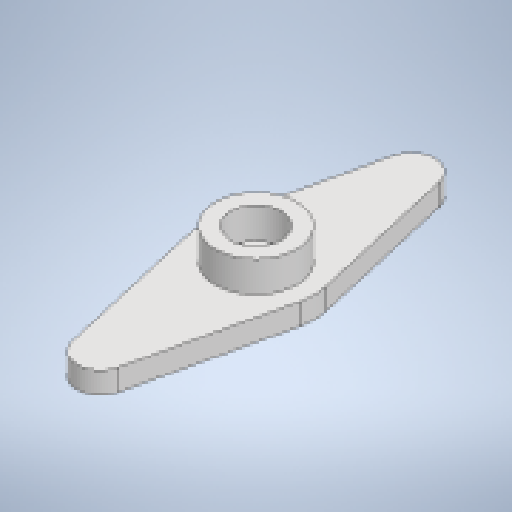
# Autodesk Inventor part: Brazo
Saved by Autodesk Inventor 2024 (Build 280153000, 153)
## iProperties
Created: 2025-03-01
Part Number: Brazo
Material: Genérico
Document SubType Name: Modeling
Designer: sergi
Density: 1 g/cm^3
Appearance: Valor por defecto
Author: sergi
Autodesk Inventor part; units mm, degrees
ref_plane "YZ Plane" through (0, 0, 0) normal (1, 0, 0) x (0, 1, 0)
ref_plane "XZ Plane" through (0, 0, 0) normal (0, 1, 0) x (-1, 0, 0)
ref_plane "XY Plane" through (0, 0, 0) normal (0, 0, 1) x (1, 0, 0)
sketch "Boceto1" plane through (0, 0, 0) normal (0, 1, 0) x (-1, 0, 0)
  circle A0 centre (0, 0) radius 1.55
  line L0 (0, 0) -> (0, -1.55)
  line L1 (0, -19.075) -> (0, -14.075)
  line L2 (0, 19.075) -> (0, 16.575)
  arc A1 (2.4369, 17.1331) -> (-2.4369, 17.1331) centre (0, 16.575) ccw
  line L3 (0, -19.075) -> (0, -16.575)
  arc A2 (-2.4369, -17.1331) -> (2.4369, -17.1331) centre (0, -16.575) ccw
  line L4 (-2.4369, 17.1331) -> (-6.0436, 1.384)
  line L5 (2.4369, 17.1331) -> (6.0436, 1.384)
  line L6 (2.4369, -17.1331) -> (6.0436, -1.384)
  line L7 (-2.4369, -17.1331) -> (-6.0436, -1.384)
  arc A3 (-6.0436, 1.384) -> (-6.0436, -1.384) centre (0, 0) ccw
  arc A4 (6.0436, -1.384) -> (6.0436, 1.384) centre (0, 0) ccw
  dimension "d0" = 3.1
  dimension "d2" = 19.075
  dimension "d3" = 38.15
  dimension "d4" = 2.5
  dimension "d5" = 2.5
  constraints: 16 end point, 11 point on circle, 8 tangent, 4 centre point, 4 coincident, 2 point on line, 1 midpoint, 1 vertical, 1 vertical alignment, 2 other
  measures "d2" distance of L0.start L1.start
  measures "d3" distance of L1.start L2.start
  measures "d4" distance of L2.start L2.end
  measures "d5" distance of L1.start L3.end
extrude "Extrusión1" add sketch "Boceto1" along normal blind 2.3
sketch "Boceto2" plane through (0, 2.3, 0) normal (0, 1, 0) x (1, 0, 0)
  circle A0 centre (0, 0) radius 1.55 projected
  circle A1 centre (0, 0) radius 4.35
  circle A2 centre (0, 0) radius 2.7
  dimension "d8" = 8.7
  dimension "d9" = 5.4
  constraints: 2 centre point, 2 coincident
  measures "d8" diameter of A1
  measures "d9" diameter of A2
extrude "Extrusión2" add sketch "Boceto2" along normal blind 3.3 contours A1
sketch "Boceto3" plane through (0, 0, 0) normal (0, -1, 0) x (1, 0, 0)
  circle A0 centre (0, 0) radius 1.55 projected
  line L0 (0, -1.55) -> (0, 1.55)
  constraints: 2 end point, 2 point on circle, 1 vertical
